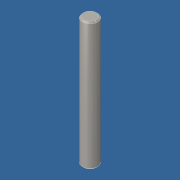
# Autodesk Inventor part: Welle_wrist
Saved by Autodesk Inventor 2016 (Build 200138000, 138)
## iProperties
Created: 2015-10-04
Part Number: Welle_wrist
Material: Edelstahl
Document SubType Name: Modeling
Designer: 4ndreas
Density: 8 g/cm^3
Appearance: Halbpoliert
Mass: 11.2819 g
Surface Area: 9.97357 cm^2
Volume: 1.41024 cm^3
Author: 4ndreas
Autodesk Inventor part; units mm, degrees
ref_plane "YZ Plane" through (0, 0, 0) normal (1, 0, 0) x (0, 1, 0)
ref_plane "XZ Plane" through (0, 0, 0) normal (0, 1, 0) x (-1, 0, 0)
ref_plane "XY Plane" through (0, 0, 0) normal (0, 0, 1) x (1, 0, 0)
sketch "Skizze1" plane through (0, 0, 0) normal (0, 0, 1) x (1, 0, 0)
  circle A0 centre (0, 0) radius 3
  dimension "d0" = 6
  constraints: 1 centre point, 1 coincident
  measures "d0" diameter of A0
extrude "Extrusion1" add sketch "Skizze1" along normal blind 8.5
sketch "Skizze2" plane through (0, 0, 8.5) normal (0, 0, 1) x (1, 0, 0)
  circle A0 centre (0, 0) radius 3 projected
  line L0 (-2.5, 1.6583) -> (-2.5, -1.6583)
  dimension "d3" = 2.5
  constraints: 2 end point, 2 point on circle, 1 vertical
  measures "d3" distance from line of L0 A0.centre
extrude "Extrusion2" add sketch "Skizze2" along normal blind 6 contours A0 L0 picked at (-0.6667, 0)
sketch "Skizze3" plane through (0, 0, 14.5) normal (0, 0, 1) x (1, 0, 0)
  circle A0 centre (0, 0) radius 3 projected
extrude "Extrusion3" add sketch "Skizze3" along normal blind 30
sketch "Skizze4" plane through (0, 0, 44.5) normal (0, 0, 1) x (1, 0, 0)
  line L0 (-2.5, -1.6583) -> (-2.5, 1.6583) projected
  arc A0 (-2.5, 1.6583) -> (-2.5, -1.6583) centre (0, 0) ccw projected
  circle A1 centre (0, 0) radius 3 projected
extrude "Extrusion4" add sketch "Skizze4" along normal blind 6 contours L0 A1
chamfer "Fase1" distance 0.5 angle 45 3 edges at (-3, 0, 0) (0.866, -2.8723, 50.5) (0.866, 2.8723, 50.5)
